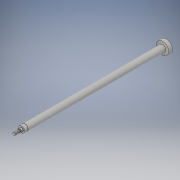
# Autodesk Inventor part: 1470874 EPCO-25-300_k---(1_0)
Saved by Autodesk Inventor 2019 (Build 230136000, 136)
## iProperties
Created: 2023-04-07
Part Number: 1470874 EPCO-25-300_k---(1_0)
Material: Generic
Catalog Web Link: www.cadenas.de
Description: EPCO_k-Piston rod
Vendor: FESTO
Document SubType Name: Modeling
Designer: psAdmin
Manufacturer: FESTO
Mass: 100.324 g
Surface Area: 242.984 cm^2
Volume: 100.324 cm^3
Density: 1 g/cm^3
Appearance: PSOLRGB-175-175-175
Category: PARTsolutions
Company: FESTO
Title: 1470874 EPCO-25-300_k---(1_0)
Author: Cadenas PARTsolutions
Comments: Piston rod
PSOL_IDENT_0: {$CADENAS_DATA/23d-libs/festo/parts/e/epco/parts/epco_k.prj},222 {VTYP=3D},{NB=1470874 EPCO-25-300_k
PSOL_IDENT_1: ---(1_0)},{LINA=1470874 EPCO-25-300_k---(1_0)},{NN=EPCO_k},{DATE=16.03.2023 11:34:06},{GEOMDATE=16.0
PSOL_IDENT_2: 3.2023 11:30:21},{VERSION=},{LINEID=20},{WBVAR=HUB,KOL,KOLB},{WBNUMERIC=HUB,KOL,KOLB}  {NB=1470874 E
PSOL_IDENT_3: PCO-25-300_k---(1_0)},{LINA=1470874 EPCO-25-300_k---(1_0)},{KT=DUMMY},{TNR=1470874},{TYP=EPCO-25},{K
PSOL_IDENT_4: DM=25},{HUB=300},{KOL=1},{KOLB=0},{L4=18.000},{D1=17.270},{D2=10.000},{AM=16.000},{L5=4.200},{SW1=9.
PSOL_IDENT_5: 000},{SW2=13.000},{KKN=8.000},{KKP=0.000},{L2=156.600},{LK=62.600},{KK1N=6.000},{KKL1=3.200},{KKL2=1
PSOL_IDENT_6: .500},{D5=6.400},{KFN=6.000},{T5=2.600},{AF=12.000}
NB: 1470874 EPCO-25-300_k---(1_0)
NN: EPCO_k
NT: Piston rod
NBSYN: $TNR. $TYP.-$HUB._k---($KOL._$KOLB.)
LINA: 1470874 EPCO-25-300_k---(1_0)
CATALOG: Festo
TNR: 1470874
TYP: EPCO-25
KDM: 25
HUB: 300
KOL: 1
KOLB: 0
L4: 18
D1: 17.27
D2: 10
AM: 16
L5: 4.2
SW1: 9
SW2: 13
KKN: 8
KKP: 0
L2: 156.6
LK: 62.6
KK1N: 6
KKL1: 3.2
KKL2: 1.5
D5: 6.4
KFN: 6
T5: 2.6
AF: 12
SUPPLIER: FESTO
ARTICLENO: 1470874 EPCO-25-300_k---(1_0)
BOMINFO: 1470874 EPCO-25-300_k---(1_0)
CREATOR: CADENAS GmbH
Autodesk Inventor part; units mm, degrees
sketch "Sketch_1" plane through (0, 0, 0) normal (1, 0, 0) x (0, 1, 0)
  line L0 (0, -384) -> (0, 18)
  line L1 (0, 18) -> (4.8, 18)
  line L2 (4.8, 18) -> (5, 17.8)
  line L3 (5, 17.8) -> (5, 13.2)
  arc A0 (5, 13.2) -> (5.4, 12.8) centre (5.4, 13.2) ccw
  line L4 (5.4, 12.8) -> (8.035, 12.8)
  line L5 (8.035, 12.8) -> (8.335, 12.5)
  line L6 (8.335, 12.5) -> (8.335, 3.1)
  arc A1 (8.335, 3.1) -> (8.635, 2.8) centre (8.635, 3.1) ccw
  line L7 (8.635, 2.8) -> (8.635, -374)
  line L8 (8.635, -374) -> (16.6667, -374)
  line L9 (16.6667, -374) -> (16.6667, -384)
  line L10 (16.6667, -384) -> (0, -384)
  line L11 (0, -384) -> (0, 18)
  constraints: 24 end point, 4 point on circle, 2 centre point
revolve "Revolution1" add sketch "Sketch_1" angle 360 about axis through (0, 0, -384) along (0, 0, -1)
sketch "Sketch_3" plane through (0, 0, 0) normal (1, 0, 0) x (0, 1, 0)
  line L0 (0, 18) -> (0, 34)
  line L1 (0, 34) -> (3.233, 34)
  line L2 (3.233, 34) -> (4, 33.233)
  line L3 (4, 33.233) -> (4, 20.8321)
  line L4 (4, 20.8321) -> (3.0804, 19.2392)
  arc A0 (3.0804, 19.2392) -> (3, 18.9392) centre (3.6, 18.9392) ccw
  line L5 (3, 18.9392) -> (3, 18.6)
  arc A1 (3, 18.6) -> (3.6, 18) centre (3.6, 18.6) ccw
  line L6 (3.6, 18) -> (0, 18)
  line L7 (0, 18) -> (0, 34)
  constraints: 16 end point, 4 point on circle, 2 centre point
revolve "Revolution2" add sketch "Sketch_3" angle 360 about axis through (0, 0, 18) along (0, 0, -1)
thread "Thread1" size "M8x1.25" class "6g" standard "ISO Metric profile" full length
sketch "Sketch_2" plane through (0, 0, 18) normal (0, 0, 1) x (1, 0, 0)
  line L0 (-6.5, 7) -> (-6.5, -5)
  line L1 (-6.5, -5) -> (-4.5, -5)
  line L2 (-4.5, -5) -> (-4.5, 5)
  line L3 (-4.5, 5) -> (4.5, 5)
  line L4 (4.5, 5) -> (4.5, -5)
  line L5 (4.5, -5) -> (6.5, -5)
  line L6 (6.5, -5) -> (6.5, 7)
  line L7 (6.5, 7) -> (-6.5, 7)
  constraints: 16 end point
extrude "Extrusion1" cut sketch "Sketch_2" against normal blind 4.2
ref_plane "EAGF_XY" through (0, 0, 18) normal (0, 0, -1) x (1, 0, 0)
ref_plane "EAGF_YZ" through (0, 0, 18) normal (1, 0, 0) x (0, -1, 0)
ref_plane "EAGF_ZX" through (0, 0, 18) normal (0, -1, 0) x (0, 0, -1)
ref_plane "EPCO_KS_XY" through (0, 0, 0) normal (0, 0, -1) x (1, 0, 0)
ref_plane "EPCO_KS_YZ" through (0, 0, 0) normal (1, 0, 0) x (0, -1, 0)
ref_plane "EPCO_KS_ZX" through (0, 0, 0) normal (0, -1, 0) x (0, 0, -1)
ref_plane "NUT_XY" through (0, 0, 26) normal (0, 0, -1) x (1, 0, 0)
ref_plane "NUT_YZ" through (0, 0, 26) normal (1, 0, 0) x (0, -1, 0)
ref_plane "NUT_ZX" through (0, 0, 26) normal (0, -1, 0) x (0, 0, -1)
body "Solid1"
